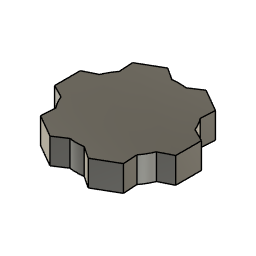
Gear_6 (Autodesk Fusion 360 design; units mm, degrees)
Autodesk Fusion 360 part; units mm, degrees
sketch "スケッチ1" plane through (0, 0, 0) normal (0, 0, 1) x (1, 0, 0)
  line L0 (-2354.0496, 500) -> (-2354.0496, -500)
  line L1 (-1854.0496, -750) -> (-1854.0496, 750) construction
  line L2 (-1854.0496, 750) -> (-2354.0496, 500)
  line L3 (-1854.0496, -750) -> (-2354.0496, -500)
  line L4 (-1610.0375, -1788.6668) -> (-744.0121, -2288.6668)
  line L5 (-277.5058, -1980.6541) -> (-1576.5439, -1230.6541) construction
  line L6 (-1576.5439, -1230.6541) -> (-1610.0375, -1788.6668)
  line L7 (-277.5058, -1980.6541) -> (-744.0121, -2288.6668)
  line L8 (744.0121, -2288.6668) -> (1610.0375, -1788.6668)
  line L9 (1576.5439, -1230.6541) -> (277.5058, -1980.6541) construction
  line L10 (277.5058, -1980.6541) -> (744.0121, -2288.6668)
  line L11 (1576.5439, -1230.6541) -> (1610.0375, -1788.6668)
  line L12 (2354.0496, -500) -> (2354.0496, 500)
  line L13 (1854.0496, 750) -> (1854.0496, -750) construction
  line L14 (1854.0496, -750) -> (2354.0496, -500)
  line L15 (1854.0496, 750) -> (2354.0496, 500)
  line L16 (1610.0375, 1788.6668) -> (744.0121, 2288.6668)
  line L17 (277.5058, 1980.6541) -> (1576.5439, 1230.6541) construction
  line L18 (1576.5439, 1230.6541) -> (1610.0375, 1788.6668)
  line L19 (277.5058, 1980.6541) -> (744.0121, 2288.6668)
  line L20 (-744.0121, 2288.6668) -> (-1610.0375, 1788.6668)
  line L21 (-1576.5439, 1230.6541) -> (-277.5058, 1980.6541) construction
  line L22 (-277.5058, 1980.6541) -> (-744.0121, 2288.6668)
  line L23 (-1576.5439, 1230.6541) -> (-1610.0375, 1788.6668)
  arc A0 (-1576.5439, 1230.6541) -> (-1854.0496, 750) centre (0, 0) ccw
  arc A1 (277.5058, 1980.6541) -> (-277.5058, 1980.6541) centre (0, 0) ccw
  arc A2 (1854.0496, 750) -> (1576.5439, 1230.6541) centre (0, 0) ccw
  arc A3 (1576.5439, -1230.6541) -> (1854.0496, -750) centre (0, 0) ccw
  arc A4 (-1854.0496, -750) -> (-1576.5439, -1230.6541) centre (0, 0) ccw
  arc A5 (-277.5058, -1980.6541) -> (277.5058, -1980.6541) centre (0, 0) ccw
  dimension "d16" = 500
  dimension "d18" = 2000
  dimension "d19" = 1000
  dimension "d20" = 1500
  dimension "d22" = 360
  constraint coincident A0.centre A1.centre
  constraint vertical L0
  constraint vertical L1
  constraint equal L2 L3
  constraint concentric A0 A4
  constraint concentric A1 A4
  constraint concentric A2 A4
  constraint concentric A3 A4
  constraint concentric A4 A5
  measures "d16" distance of L0 L1
  measures "d18" radius of A4
  measures "d19" distance of L0.start L0.end
  measures "d20" distance of L1.end L1.start
extrude "押し出し1" add sketch "スケッチ1" along normal blind 1000
